Autodesk Inventor part; units mm, degrees
(part 3 of 3)
extrude "Extrusion10" cut sketch "Sketch10" against normal blind 78.74 contours L71 L87 L90 L89 | L71 L83 L86 L85 | L75 L78 L77 L71 | L71 L79 L82 L81
fillet "Fillet2" radius 5.08 25 edges at (-0.4003, 36.83, -44.8035) (-20.522, 0, -44.8035) (-0.4003, 0, -50.8) (-11.0395, 0, -56.7965) (-0.4003, 36.83, -56.7965) (-0.4003, 36.83, -18.9452) (-20.522, 0, -18.9452) (-0.4003, 0, -25.4) (-20.522, 0, -31.8548) (-0.4003, 36.83, -31.8548) (-20.522, 0, -6.2347) (-0.4003, 0, 0) (-0.4003, 36.83, -6.2347) (-0.4003, 36.83, 6.2347) (-20.522, 0, 6.2347) (-20.522, 0, 18.8766) (-0.4003, 36.83, 18.8766) (-0.4003, 0, 25.4) (-0.4003, 36.83, 31.9234) (-20.522, 0, 31.9234) (-20.522, 0, 43.6993) (-0.4003, 0, 50.8) (-9.899, 0, 57.9007) (-0.4003, 36.83, 43.6993) (-0.4003, 36.83, 57.9007)
fillet "Fillet3" radius 5.08 16 edges at (-40.6438, 1.4879, -46.2914) (-40.6438, 41.91, -44.8035) (-40.6438, 1.4879, -20.4331) (-40.6438, 41.91, -18.9452) (-40.6438, 1.4879, 4.7468) (-40.6438, 41.91, 6.2347) (-40.6438, 1.4879, 30.4355) (-40.6438, 41.91, 31.9234) (-40.6438, 1.4879, 20.3645) (-40.6438, 41.91, 18.8766) (-40.6438, 1.4879, -4.7468) (-40.6438, 41.91, -6.2347) (-40.6438, 1.4879, -30.3669) (-40.6438, 41.91, -31.8548) (-40.6438, 1.4879, 45.1872) (-40.6438, 41.91, 43.6993)
equation "\"d3\" = d2"
equation "\"d19\" = d18"
equation "\"d20\" = d18"
equation "\"d22\" = d18"
equation "\"d39\" = d38"
equation "\"d40\" = d38"
equation "\"d41\" = d38"
equation "\"d42\" = d41"
equation "\"d43\" = d40"
equation "\"d49\" = d46"
equation "\"d53\" = d52"
equation "\"d54\" = d52"
equation "\"d55\" = d53"
equation "\"d56\" = d55"
equation "\"d57\" = d56"
equation "\"d58\" = d57"
equation "\"d59\" = d58"
equation "\"d60\" = d59"
body "Solid1"
